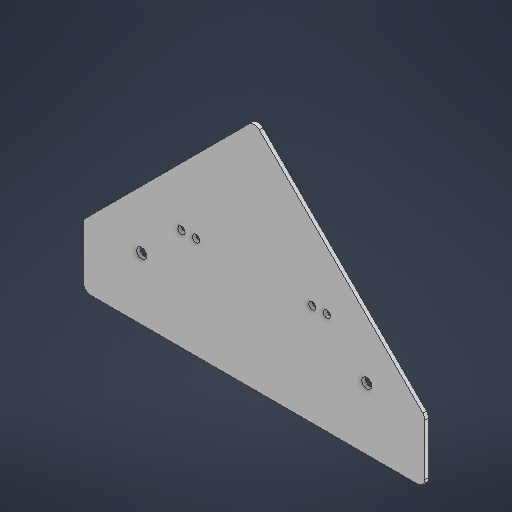
# Autodesk Inventor part: alignernew
Saved by Autodesk Inventor 2026.1 (Build 301233000, 233)
## iProperties
Created: 2026-01-08
Part Number: alignernew
Material: Generic
Document SubType Name: Modeling
Designer: roejo
Density: 1 g/cm^3
Appearance: Default
Author: roejo
Autodesk Inventor part; units mm, degrees
ref_plane "YZ Plane" through (0, 0, 0) normal (1, 0, 0) x (0, 1, 0)
ref_plane "XZ Plane" through (0, 0, 0) normal (0, 1, 0) x (-1, 0, 0)
ref_plane "XY Plane" through (0, 0, 0) normal (0, 0, 1) x (1, 0, 0)
sketch "Sketch1" plane through (0, 0, 0) normal (0, 0, 1) x (1, 0, 0)
  arc A0 (145.923, -27.051) -> (149.098, -23.876) centre (145.923, -23.876) ccw
  circle A1 centre (49.149, 17.399) radius 1.5875
  line L0 (149.098, -1.3151) -> (149.098, -23.876)
  line L1 (0, -23.876) -> (0, -1.3151)
  circle A2 centre (106.299, 17.399) radius 1.5875
  line L2 (148.1681, 0.9299) -> (76.7941, 72.3039)
  line L3 (0.9299, 0.9299) -> (72.3039, 72.3039)
  circle A3 centre (42.799, 17.399) radius 1.5875
  circle A4 centre (25.4, 0) radius 2.2098
  circle A5 centre (123.698, 0) radius 2.2098
  arc A6 (0, -23.876) -> (3.175, -27.051) centre (3.175, -23.876) ccw
  arc A7 (76.7941, 72.3039) -> (72.3039, 72.3039) centre (74.549, 70.0589) ccw
  arc A8 (0.9299, 0.9299) -> (0, -1.3151) centre (3.175, -1.3151) ccw
  circle A9 centre (99.949, 17.399) radius 1.5875
  arc A10 (149.098, -1.3151) -> (148.1681, 0.9299) centre (145.923, -1.3151) ccw
  line L4 (74.549, 73.2339) -> (74.549, -27.051)
  line L5 (145.923, -27.051) -> (3.175, -27.051)
  point P0 (0, 0)
  point P1 (76.7941, 72.3039)
  point P2 (0, -1.3151)
  point P3 (74.549, 23.0914)
  point P4 (3.175, -27.051)
  dimension "d2" = 6.35
  dimension "d3" = 6.35
  dimension "d4" = 25.4
  dimension "d5" = 25.4
  dimension "d8" = 44.45
  dimension "d9" = 44.45
  constraints: 12 end point, 11 centre point, 11 point on circle, 1 midpoint
  measures "d2" distance of A3.centre A1.centre
  measures "d3" distance of A2.centre A9.centre
  measures "d4" horizontal distance of point (74.549, 23.091) A1.centre
  measures "d5" distance from line of L4 A9.centre
  measures "d8" distance from line of L5 A1.centre
  measures "d9" distance from line of L5 A9.centre
extrude "Extrusion1" add sketch "Sketch1" along normal blind 1.5875
body "Solid1"
